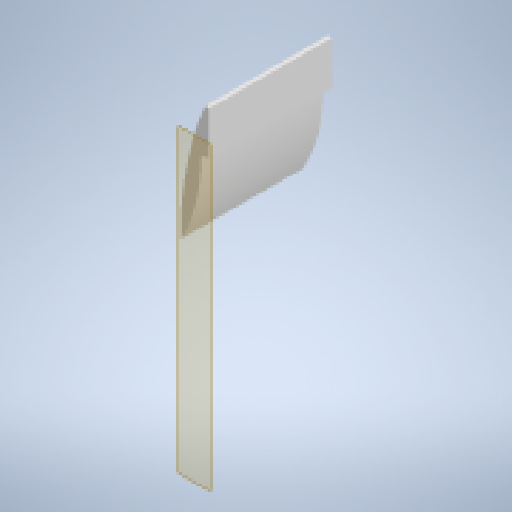
# Autodesk Inventor part: WingBox
Saved by Autodesk Inventor 2026 (Build 300175050, 175E)
## iProperties
Created: 2025-08-01
Part Number: WingBox
Material: Plastic, Opaque White
Document SubType Name: Modeling
Designer: Cupri
Mass: 728.648 g
Surface Area: 2482.51 cm^2
Volume: 765.387 cm^3
Density: 0.952 g/cm^3
Appearance: Smooth - White
Author: Cupri
Autodesk Inventor part; units mm, degrees
ref_plane "YZ Plane" through (0, 0, 0) normal (1, 0, 0) x (0, 1, 0)
ref_plane "XZ Plane" through (0, 0, 0) normal (0, 1, 0) x (-1, 0, 0)
ref_plane "XY Plane" through (0, 0, 0) normal (0, 0, 1) x (1, 0, 0)
ref_plane "Work Plane1" through (0, 0, 0) normal (0, 0, 1) x (1, 0, 0)
sketch "Sketch1" plane through (0, 0, 0) normal (0, 0, 1) x (1, 0, 0)
  line L0 (17.5439, 167.3777) -> (17.5439, -167.2177)
  line L1 (12.6198, 167.3777) -> (17.5439, 167.3777)
  arc A0 (12.6198, 167.3777) -> (7.6198, 162.3647) centre (12.6198, 162.3777) ccw
  arc A1 (-17.2206, 65.3053) -> (7.6198, 162.3647) centre (-192.3795, 161.842) ccw
  spline S0 degree 3 poles (15.5066, -167.3777) (14.148, -162.3458) (13.1454, -158.733) (12.2209, -155.3522) (11.2937, -151.9614) (10.4451, -148.804) (9.5187, -145.1939) (8.5922, -141.5836) (7.5879, -137.5207) (6.4718, -132.8251) (5.3468, -128.0919) (4.108, -122.7149) (2.8468, -117.0311) (1.5537, -111.2034) (0.2595, -105.1403) (-0.9267, -99.2767) (-2.1322, -93.3183) (-3.2259, -87.5664) (-4.2378, -81.9453) (-5.5682, -74.5555) (-6.7904, -67.2856) (-7.9716, -59.8366) (-9.5523, -49.8682) (-11.0261, -39.597) (-12.2642, -29.3514) (-13.1409, -22.0968) (-13.9086, -14.884) (-14.597, -7.8525) (-15.2681, -0.9965) (-15.8677, 5.6744) (-16.3523, 12.5437) (-16.7137, 17.6683) (-17.0046, 22.9717) (-17.2019, 28.5104) (-17.3991, 34.0437) (-17.5029, 39.8119) (-17.5246, 45.3475) (-17.5439, 50.2823) (-17.5013, 54.9542) (-17.4101, 59.0831) (-17.3611, 61.3015) (-17.298, 63.3631) (-17.2206, 65.3053) knots 0 0 0 0 0.065999 0.065999 0.065999 0.132191 0.132191 0.132191 0.198388 0.198388 0.198388 0.265115 0.265115 0.265115 0.33353 0.33353 0.33353 0.403053 0.403053 0.403053 0.494451 0.494451 0.494451 0.616763 0.616763 0.616763 0.703369 0.703369 0.703369 0.787814 0.787814 0.787814 0.850812 0.850812 0.850812 0.913749 0.913749 0.913749 0.969854 0.969854 0.969854 1 1 1 1
  line L2 (16.0762, -167.2239) -> (15.5066, -167.3777)
  line L3 (17.2649, -167.2189) -> (16.0762, -167.2239)
  line L4 (17.2649, -167.2177) -> (17.2649, -167.2189)
  line L5 (17.5439, -167.2177) -> (17.2649, -167.2177)
  line L6 (-7.3809, 65.3274) -> (-7.2942, 45.0687)
  line L7 (12.9046, 65.3964) -> (-7.3809, 65.3274)
  line L8 (12.9735, 45.1555) -> (12.9046, 65.3964)
  line L9 (-7.2942, 45.0687) -> (12.9735, 45.1555)
  arc A2 (12.5439, 221.0296) -> (-17.2206, 65.3053) centre (374.4763, 71.1448) ccw
  line L10 (12.5439, 221.0296) -> (17.5439, 221.0296)
  line L11 (17.5439, 221.0296) -> (17.5439, 167.3777)
  line L12 (17.5439, 167.3777) -> (12.6198, 167.3777)
  point P0 (0, 0)
  dimension "d0" = 5
  constraints: 6 end point, 3 point on circle, 1 centre point, 1 horizontal, 1 parallel, 1 perpendicular
  measures "d0" distance of L10.start L10.end
extrude "Extrusion1" add sketch "Sketch1" against normal blind 150 contours L1 A0 A1 A2 L10 L11
sketch "Sketch2" plane through (12.5439, 221.0296, 0) normal (0, 1, 0) x (1, 0, 0)
  line L0 (0.0759, 0) -> (-4.9241, 0) projected
  line L1 (0.0759, 0) -> (125.0759, 0)
  line L2 (125.0759, 0) -> (125.0759, 150)
  line L3 (125.0759, 150) -> (0.0759, 150)
  line L4 (0.0759, 150) -> (0.0759, 0)
  line L5 (5, 0) -> (5, 150) projected
  line L6 (5, 2.5) -> (117.0759, 2.5)
  line L7 (117.0759, 2.5) -> (117.0759, 147.5)
  line L8 (117.0759, 147.5) -> (5, 147.5)
  line L9 (5, 147.5) -> (5, 2.5)
  point P0 (-12.5439, 0)
  point P1 (-4.9241, 0)
  point P2 (5, 147.5)
  dimension "d3" = 125
  dimension "d4" = 2.5
  dimension "d5" = 2.5
  dimension "d6" = 8
  constraints: 16 end point, 4 parallel, 2 horizontal, 2 perpendicular, 1 point on line
  measures "d3" distance of L3.end L2.end
  measures "d4" distance between parallel lines of L1 L6
  measures "d5" distance between parallel lines of L3 L8
  measures "d6" distance between parallel lines of L2 L7
extrude "Extrusion2" add sketch "Sketch2" against normal blind 250 contours L5 L6 L7 L8 L3 L2 L1
body "Solid1"
